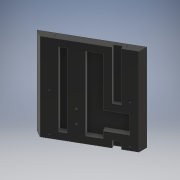
# Autodesk Inventor part: HB02
Saved by Autodesk Inventor 2017 (Build 210142000, 142)
## iProperties
Created: 2019-05-20
Part Number: HB02
Material: Polyethylene, High Density
Document SubType Name: Modeling
Designer: Dell
Density: 0.952 g/cm^3
Appearance: Smooth - Black
Mass: 1766.71 g
Surface Area: 2613.22 cm^2
Volume: 1855.79 cm^3
Author: Dell
Autodesk Inventor part; units mm, degrees
ref_plane "YZ Plane" through (0, 0, 0) normal (1, 0, 0) x (0, 1, 0)
ref_plane "XZ Plane" through (0, 0, 0) normal (0, 1, 0) x (-1, 0, 0)
ref_plane "XY Plane" through (0, 0, 0) normal (0, 0, 1) x (1, 0, 0)
sketch "Sketch1" plane through (0, 0, 0) normal (0, 0, 1) x (1, 0, 0)
  line L0 (262.89, 151.7796) -> (525.78, 0) construction
  line L1 (525.78, 0) -> (525.78, -303.5592) construction
  line L2 (525.78, -303.5592) -> (262.89, -455.3388) construction
  line L3 (262.89, -455.3388) -> (0, -303.5592) construction
  line L4 (0, -303.5592) -> (0, 0) construction
  line L5 (0, 0) -> (262.89, 151.7796)
  line L6 (0, 0) -> (25.4, -14.6647)
  line L7 (25.4, -14.6647) -> (262.89, 122.4502)
  line L8 (262.89, 122.4502) -> (262.89, 151.7796)
  point P0 (262.89, -151.7796)
  dimension "d0" = 525.78
  dimension "d2" = 25.4
  dimension "d3" = 60
  dimension "d4" = 60
  constraints: 18 end point, 1 coincident, 1 parallel, 1 vertical, 13 other
  measures "d0" distance between parallel lines of L1 L4
  measures "d2" distance between parallel lines of L5 L7
  measures "d3" angle of L5 L8
  measures "d4" angle of L5 L6
extrude "Extrusion1" add sketch "Sketch1" along normal blind 330.2
sketch "Sketch8" plane through (0, 0, 0) normal (0, 0, -1) x (-1, 0, 0)
  line L0 (-25.4, -14.6647) -> (-262.89, 122.4502) projected
  line L1 (-198.618, 85.3428) -> (-192.268, 96.3413)
  line L2 (-192.268, 96.3413) -> (-214.265, 109.0413)
  line L3 (-214.265, 109.0413) -> (-220.615, 98.0428)
  line L4 (-198.618, 85.3428) -> (-220.615, 98.0428)
  point P0 (0, 0)
  dimension "d47" = 25.4
  dimension "d48" = 12.7
  dimension "d49" = 48.8149
  constraints: 8 end point, 3 perpendicular, 2 point on line, 1 collinear
  measures "d47" distance of L1.end L2.end
  measures "d48" distance of L1.start L1.end
  measures "d49" distance from line of L0.end L3
extrude "Extrusion7" cut sketch "Sketch8" against normal blind 25.4
sketch "Sketch9" plane through (0, 0, 330.2) normal (0, 0, 1) x (1, 0, 0)
  line L0 (192.268, 96.3413) -> (198.618, 85.3428) projected
  line L1 (214.265, 109.0413) -> (192.268, 96.3413) projected
  line L2 (220.615, 98.0428) -> (214.265, 109.0413) projected
  line L3 (198.618, 85.3428) -> (220.615, 98.0428) projected
  point P0 (0, 0)
extrude "Extrusion8" cut sketch "Sketch9" against normal blind 185
sketch "Sketch10" plane through (25.4, -14.6647, 0) normal (0.5, -0.8660254, 0) x (0.8660254, 0.5, 0)
  line L0 (25.4, 157.9) -> (248.8298, 157.9) construction
  line L1 (248.8298, 157.9) -> (248.8298, 12.7) construction
  line L2 (248.8298, 12.7) -> (25.4, 12.7) construction
  line L3 (25.4, 12.7) -> (25.4, 157.9) construction
  line L4 (225.4149, 145.2) -> (200.0149, 145.2) construction
  line L5 (200.0149, 25.4) -> (225.4149, 25.4) construction
  line L6 (274.2298, 0) -> (274.2298, 330.2) construction
  line L7 (0, 0) -> (0, 330.2) construction
  circle A0 centre (25.4, 157.9) radius 2
  circle A1 centre (25.4, 12.7) radius 2
  circle A2 centre (248.8298, 157.9) radius 2
  circle A3 centre (248.8298, 12.7) radius 2
  point P0 (-14.6647, 0)
  dimension "d54" = 12.7
  dimension "d55" = 12.7
  dimension "d56" = 25.4
  dimension "d57" = 25.4
  dimension "d58" = 4
  dimension "d59" = 4
  dimension "d60" = 4
  dimension "d61" = 4
  constraints: 8 end point, 4 centre point, 4 coincident, 2 parallel, 1 horizontal, 1 perpendicular
  measures "d54" distance between parallel lines of L4 L0
  measures "d55" distance between parallel lines of L5 L2
  measures "d56" distance between parallel lines of L6 L1
  measures "d57" distance between parallel lines of L7 L3
  measures "d58" diameter of A0
  measures "d59" diameter of A1
  measures "d60" diameter of A2
  measures "d61" diameter of A3
extrude "Extrusion9" cut sketch "Sketch10" against normal through all
sketch "Sketch11" plane through (0, 0, 330.2) normal (-0.5, 0.8660254, 0) x (0.8660254, 0.5, 0)
  circle A0 centre (263.4945, 172.3) radius 2 projected
  circle A1 centre (263.4945, 317.5) radius 2 projected
  circle A2 centre (40.0647, 317.5) radius 2 projected
  circle A3 centre (40.0647, 172.3) radius 2 projected
  circle A4 centre (263.4945, 172.3) radius 6.5
  circle A5 centre (40.0647, 172.3) radius 2 projected
  circle A6 centre (40.0647, 172.3) radius 6.5
  circle A7 centre (40.0647, 317.5) radius 6.5
  circle A8 centre (263.4945, 317.5) radius 2 projected
  circle A9 centre (263.4945, 317.5) radius 6.5
  point P0 (0, 330.2)
  dimension "d64" = 13
  dimension "d65" = 13
  dimension "d66" = 13
  dimension "d67" = 13
  constraints: 4 centre point, 4 coincident
  measures "d64" diameter of A4
  measures "d65" diameter of A6
  measures "d66" diameter of A7
  measures "d67" diameter of A9
extrude "Extrusion10" cut sketch "Sketch11" against normal blind 12.7 contours A0 | A1 | A2 | A3 | A4 | A6 | A7 | A9
sketch "Sketch12" plane through (0, 0, 330.2) normal (-0.5, 0.8660254, 0) x (0.8660254, 0.5, 0)
  circle A0 centre (115.0647, 269.9) radius 4
  circle A1 centre (115.0647, 219.9) radius 4
  circle A2 centre (40.0647, 317.5) radius 6.5 construction
  circle A3 centre (40.0647, 172.3) radius 6.5 construction
  circle A4 centre (40.0647, 317.5) radius 2 projected
  circle A5 centre (40.0647, 172.3) radius 2 projected
  line L0 (40.0647, 317.5) -> (40.0647, 172.3) construction
  line L1 (115.0647, 269.9) -> (115.0647, 219.9) construction
  point P0 (0, 330.2)
  point P1 (40.0647, 244.9)
  point P2 (115.0647, 244.9)
  dimension "d70" = 8
  dimension "d71" = 8
  dimension "d72" = 75
  dimension "d73" = 50
  constraints: 4 end point, 2 centre point, 2 midpoint, 2 vertical, 1 horizontal alignment, 1 vertical alignment
  measures "d70" diameter of A0
  measures "d71" diameter of A1
  measures "d72" horizontal distance of A2.centre L1.start
  measures "d73" distance of L1.end L1.start
extrude "Extrusion11" cut sketch "Sketch12" against normal through all contours A0 | A1
sketch "Sketch13" plane through (0, 0, 330.2) normal (-0.5, 0.8660254, 0) x (0.8660254, 0.5, 0)
  circle A0 centre (115.0647, 219.9) radius 4 projected
  circle A1 centre (115.0647, 269.9) radius 4 projected
  circle A2 centre (115.0647, 219.9) radius 7.5
  circle A3 centre (115.0647, 269.9) radius 7.5
  point P0 (0, 330.2)
  dimension "d76" = 15
  dimension "d77" = 15
  constraints: 2 centre point, 2 coincident
  measures "d76" diameter of A2
  measures "d77" diameter of A3
extrude "Extrusion12" cut sketch "Sketch13" against normal blind 12.7 contours A0 | A1 | A2 | A3
sketch "Sketch14" plane through (25.4, -14.6647, 0) normal (0.5, -0.8660254, 0) x (0.8660254, 0.5, 0)
  line L0 (50.8, 304.8) -> (75, 304.8)
  line L1 (75, 304.8) -> (75, 25.4)
  line L2 (75, 25.4) -> (50.8, 25.4)
  line L3 (50.8, 25.4) -> (50.8, 304.8)
  line L4 (125.8, 25.4) -> (174.6149, 25.4)
  line L5 (174.6149, 25.4) -> (174.6149, 304.8)
  line L6 (174.6149, 304.8) -> (125.8, 304.8)
  line L7 (125.8, 304.8) -> (125.8, 25.4)
  line L8 (174.6149, 119.8) -> (248.8298, 119.8)
  line L9 (248.8298, 119.8) -> (248.8298, 50.8)
  line L10 (248.8298, 50.8) -> (174.6149, 50.8)
  line L11 (174.6149, 50.8) -> (174.6149, 119.8)
  line L12 (0, 330.2) -> (200.0149, 330.2) projected
  line L13 (0, 0) -> (200.0149, 0) projected
  line L14 (200.0149, 0) -> (200.0149, 25.4) projected
  circle A0 centre (100.4, 110.3) radius 4 projected
  circle A1 centre (25.4, 157.9) radius 2 projected
  line L15 (225.4149, 145.2) -> (200.0149, 145.2) projected
  line L16 (200.0149, 25.4) -> (225.4149, 25.4) projected
  line L17 (274.2298, 0) -> (274.2298, 330.2) projected
  point P0 (-14.6647, 0)
  dimension "d80" = 25.4
  dimension "d81" = 25.4
  dimension "d82" = 25.4
  dimension "d83" = 25.4
  dimension "d84" = 25.4
  dimension "d85" = 25.4
  dimension "d86" = 25.4
  dimension "d87" = 25.4
  dimension "d88" = 25.4
  constraints: 24 end point, 6 parallel, 3 horizontal, 3 perpendicular, 2 point on line, 1 horizontal alignment
  measures "d80" distance between parallel lines of L12 L0
  measures "d81" distance between parallel lines of L13 L2
  measures "d82" distance between parallel lines of L14 L5
  measures "d83" distance from line of L7 A0.centre
  measures "d84" distance from line of L1 A0.centre
  measures "d85" distance from line of A1.centre L3
  measures "d86" distance between parallel lines of L8 L15
  measures "d87" distance between parallel lines of L16 L10
  measures "d88" distance between parallel lines of L9 L17
extrude "Extrusion13" cut sketch "Sketch14" against normal blind 19.05 contours L0 L1 L2 L3 | L7 L6 L5 L4 | L5 L8 L9 L10
sketch "Sketch15" plane through (0, 0, 330.2) normal (0, 0, 1) x (1, 0, 0)
  line L0 (12.7, -7.3323) -> (262.89, 137.1149) construction
  line L1 (0, 0) -> (25.4, -14.6647) projected
  line L2 (262.89, 122.4502) -> (262.89, 151.7796) projected
  line L3 (51.1925, 14.8913) -> (224.3975, 114.8913)
  circle A0 centre (51.1925, 14.8913) radius 2
  circle A1 centre (224.3975, 114.8913) radius 2
  point P0 (137.795, 64.8913)
  dimension "d91" = 200
  dimension "d92" = 4
  dimension "d93" = 4
  constraints: 4 end point, 4 midpoint, 2 centre point, 2 coincident, 2 point on line
  measures "d91" distance of L3.end L3.start
  measures "d92" diameter of A0
  measures "d93" diameter of A1
extrude "Extrusion14" cut sketch "Sketch15" against normal blind 38.1
body "Solid1"
